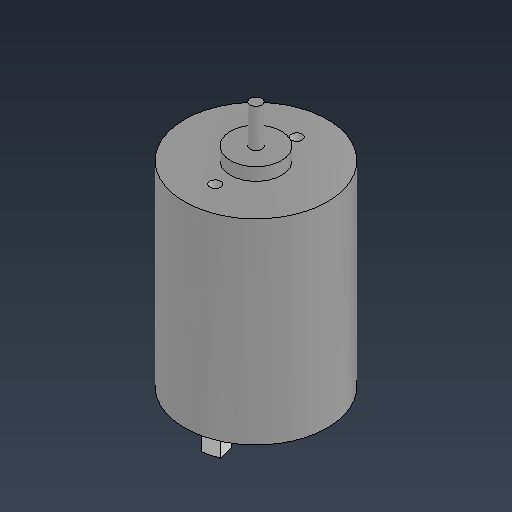
# Autodesk Inventor part: rs385
Saved by Autodesk Inventor 2026.2 (Build 302298010, 298A)
## iProperties
Created: 2025-03-30
Part Number: rs385
Material: Generic
Document SubType Name: Modeling
Designer: szymo
Density: 3.31598 g/cm^3
Appearance: Default
Mass: 80 g
Surface Area: 50.2469 cm^2
Volume: 24.1256 cm^3
Author: szymo
Autodesk Inventor part; units mm, degrees
ref_plane "YZ Plane" through (0, 0, 0) normal (1, 0, 0) x (0, 1, 0)
ref_plane "XZ Plane" through (0, 0, 0) normal (0, 1, 0) x (-1, 0, 0)
ref_plane "XY Plane" through (0, 0, 0) normal (0, 0, 1) x (1, 0, 0)
sketch "Sketch1" plane through (0, 0, 0) normal (0, 1, 0) x (-1, 0, 0)
  circle A0 centre (0, 0) radius 14
  dimension "d0" = 28
  constraints: 1 centre point, 1 coincident
  measures "d0" diameter of A0
extrude "Extrusion1" add sketch "Sketch1" along normal blind 38.4
sketch "Sketch2" plane through (0, 38.4, 0) normal (0, 1, 0) x (1, 0, 0)
  circle A0 centre (0, 0) radius 5
  circle A1 centre (0, 0) radius 1.15
  circle A2 centre (0, 0) radius 8
  line L0 (0, -8) -> (0, 8)
  dimension "d3" = 10
  dimension "d6" = 2.3
  dimension "d9" = 16
  constraints: 6 coincident, 3 centre point, 2 end point, 2 point on circle, 1 midpoint, 1 vertical
  measures "d3" diameter of A0
  measures "d6" diameter of A1
  measures "d9" diameter of A2
extrude "Extrusion2" add sketch "Sketch2" along normal blind 2.5 contours A0 L0 A1 | L0 A1 A0 | L0 A1 | A1 L0
extrude "Extrusion3" add sketch "Sketch2" along normal blind 10 contours L0 A1 | A1 L0
hole "Hole1" at (0, 38.4, 8) at (0, 38.4, -8) direction (0, -1, 0) diameter 2.1129 depth 7.8 thread size "M2.6x0.45" class "6H" standard "ISO Metric profile"
sketch "Sketch3" plane through (0, 0, 0) normal (0, -1, 0) x (1, 0, 0)
  circle A0 centre (0, 0) radius 5
  dimension "d17" = 10
  constraints: 1 centre point, 1 coincident
  measures "d17" diameter of A0
extrude "Extrusion4" add sketch "Sketch3" along normal blind 4
sketch "Sketch4" plane through (0, 0, 0) normal (0, -1, 0) x (1, 0, 0)
  line L0 (-12.0122, 7.6623) -> (12.8258, 7.6623) construction
  line L1 (12.8258, 7.6623) -> (12.8258, -7.5309) construction
  line L2 (12.8258, -7.5309) -> (-12.0122, -7.5309) construction
  line L3 (-12.0122, -7.5309) -> (-12.0122, 7.6623) construction
  point P0 (0, 0)
  constraints: 2 other
sketch "Sketch5" plane through (0, 0, 0) normal (0, -1, 0) x (1, 0, 0)
  circle A0 centre (0, 8) radius 1.0564 projected
  circle A1 centre (0, -8) radius 1.0564 projected
  circle A2 centre (0, 0) radius 5 projected
  circle A3 centre (0, 0) radius 14 projected
  circle A4 centre (0, 0) radius 1.15 projected
  circle A5 centre (0, 0) radius 12.5
  circle A6 centre (0, 0) radius 9.5
  line L0 (4.6607, 11.5986) -> (3.8768, 8.673)
  line L1 (1.763, 12.3751) -> (0.979, 9.4494)
  line L2 (-0.979, -9.4494) -> (-1.763, -12.3751)
  line L3 (-3.8768, -8.673) -> (-4.6607, -11.5986)
  line L4 (3.6235, 13.523) -> (-3.6235, -13.523)
  line L5 (0, 14) -> (0, -14) construction
  circle A7 centre (0, 0) radius 14 projected
  dimension "d21" = 3
  dimension "d27" = 19
  dimension "d28" = 1.5
  dimension "d29" = 15
  dimension "d30" = 1.5
  dimension "d31" = 1.5
  dimension "d32" = 1.5
  dimension "d33" = 1.5
  constraints: 12 end point, 12 point on circle, 3 parallel, 2 centre point, 2 coincident, 2 point on line, 1 midpoint, 1 vertical
  measures "d21" radial gap between concentric circles of A5 A6
  measures "d27" diameter of A6
  measures "d28" radial gap between concentric circles of A3 A5
  measures "d29" angle of L5 L4
  measures "d30" distance between parallel lines of L0 L4
  measures "d31" distance between parallel lines of L4 L1
  measures "d32" distance between parallel lines of L2 L4
  measures "d33" distance between parallel lines of L4 L3
extrude "Extrusion5" add sketch "Sketch5" along normal up to surface (4 mm away) contours L4 A5 L0 A6 | A6 L1 A5 L4 | L4 A5 L3 A6 | A6 L2 A5 L4
equation "\"d31\" = d30"
equation "\"d32\" = d30"
body "Solid1"
